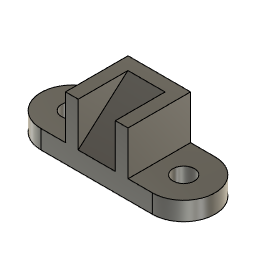
A2 piece v1 (Autodesk Fusion 360 design; units mm, degrees)
Autodesk Fusion 360 part; units mm, degrees
sketch "top view" plane through (0, 0, 0) normal (0, 0, 1) x (1, 0, 0)
  line L0 (0, 0) -> (-57, 0)
  line L1 (-57, 0) -> (-57, 64) construction
  line L2 (-57, 64) -> (0, 64)
  line L3 (0, 64) -> (0, 0) construction
  circle A0 centre (-57, 32) radius 11
  line L4 (0, 0) -> (57, 0)
  line L5 (57, 0) -> (57, 64) construction
  circle A1 centre (57, 32) radius 11
  line L6 (57, 64) -> (0, 64)
  arc A2 (-57, 64) -> (-57, 0) centre (-57, 32) ccw
  arc A3 (57, 0) -> (57, 64) centre (57, 32) ccw
  line L7 (0, 64) -> (-32, 64)
  line L8 (-32, 64) -> (-32, 0)
  line L9 (-32, 0) -> (0, 0)
  line L10 (0, 0) -> (0, 64) construction
  line L11 (32, 64) -> (32, 0)
  dimension "d1" = 64
  dimension "d2" = 57
  dimension "d3" = 22
  dimension "d4" = 0
  dimension "d5" = 32
  constraint horizontal L0
  constraint vertical L1
  constraint horizontal L2
  constraint vertical L3
  constraint coincident L0.start L3.end
  constraint midpoint L1 A0.centre
  constraint concentric A0 A2
  constraint symmetric L0.start L3 L4.start
  constraint symmetric L0.end L3 L4.end
  constraint symmetric L1.end L3 L5.end
  constraint symmetric L2.end L3 L6.end
  constraint symmetric L3 A2 A3
  constraint symmetric L3 A0 A1
  constraint horizontal L7
  constraint vertical L8
  constraint horizontal L9
  constraint vertical L10
  constraint coincident L0 L8.end
  constraint symmetric L7.end L10 L11.start
  constraint symmetric L8.end L10 L11.end
  measures "d1" distance of L0.start L2.end
  measures "d2" distance of L0.start L0.end
  measures "d3" diameter of A0
  measures "d4" distance of L2 L7
  measures "d5" distance of L2.end L7.end
extrude "Extrude1" add sketch "top view" along normal blind 19
extrude "Extrude2" add sketch "top view" along normal blind 64 contours L0 L2 L4 L6 L7 L8 L9 L11
sketch "middle part top view" plane through (0, 0, 64) normal (0, 0, 1) x (-1, 0, 0)
  line L0 (-32, -64) -> (32, -64)
  line L1 (32, -64) -> (32, 0)
  line L2 (32, 0) -> (-32, 0)
  line L3 (-32, 0) -> (-32, -64)
  line L4 (32, -64) -> (-32, -64)
  line L5 (-32, -64) -> (-32, 0)
  line L6 (-32, 0) -> (32, 0)
  line L7 (32, 0) -> (32, -64)
  line L8 (32, 0) -> (19, 0)
  line L9 (19, 0) -> (19, -51)
  line L10 (19, -51) -> (32, -51) construction
  line L11 (32, -51) -> (32, 0)
  line L12 (0, -64) -> (0, 0) construction
  line L13 (-19, 0) -> (-19, -51)
  line L14 (-19, -51) -> (-32, -51) construction
  line L15 (19, -51) -> (-19, -51)
  dimension "d11" = 51
  dimension "d12" = 13
  constraint horizontal L4
  constraint vertical L5
  constraint horizontal L6
  constraint vertical L7
  constraint coincident L2.end L3.start
  constraint coincident L0.end L1.start
  constraint horizontal L8
  constraint vertical L9
  constraint horizontal L10
  constraint vertical L11
  constraint midpoint L4 L12.start
  constraint coincident L12.end origin
  constraint symmetric L8.end L12 L13.start
  constraint symmetric L9.end L12 L13.end
  constraint symmetric L10.end L12 L14.end
  measures "d11" distance of L1.end L10.end
  measures "d12" distance of L9.end L10.end
extrude "Extrude3" cut sketch "middle part top view" against normal blind 45 contours L2 L6 L9 L13 L15
draft "Draft1" angle -41.5 neutral plane through (0, 0, 0) pull (0, 1, 0) 1 faces at (6.3333, 17, 19)
equation "d13 = -64 mm + 19.00 mm"
named bodies: "A2"
